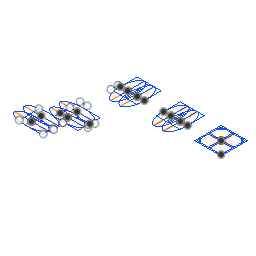
Plano_Apoyos v6 (Autodesk Fusion 360 design; units mm, degrees)
Autodesk Fusion 360 part; units mm, degrees
sketch "V1" plane through (0, 0, 0) normal (0, 1, 0) x (1, 0, 0)
  line L0 (10, -15) -> (10, -28)
  line L1 (10, -28) -> (10, -43)
  line L2 (10, -43) -> (10, -56)
  line L3 (60, -56) -> (60, -43)
  line L4 (60, -43) -> (60, -28)
  line L5 (60, -28) -> (60, -15)
  line L6 (64.9198, -28) -> (64.9198, -34)
  line L7 (64.9198, -34) -> (64.9198, -37)
  line L8 (64.9198, -37) -> (64.9198, -43)
  line L9 (60, -34) -> (35, -34)
  line L10 (35, -34) -> (35, -37)
  line L11 (35, -37) -> (60, -37)
  line L12 (60, -131, 30) -> (60, -118, 30)
  line L13 (60, -118, 30) -> (60, -103, 30)
  line L14 (60, -103, 30) -> (60, -90, 30)
  line L15 (10, -90, 30) -> (10, -103, 30)
  line L16 (10, -103, 30) -> (10, -118, 30)
  line L17 (10, -118, 30) -> (10, -131, 30)
  line L18 (60, -109, 30) -> (35, -109, 30)
  line L19 (35, -112, 30) -> (60, -112, 30)
  line L20 (35, -109, 30) -> (35, -112, 30)
  line L21 (35, -109, 30) -> (10, -109, 30)
  line L22 (35, -112, 30) -> (10, -112, 30)
  line L23 (60, -15) -> (60, -12.5)
  line L24 (60, -12.5) -> (10, -12.5)
  line L25 (10, -12.5) -> (10, -15)
  line L26 (10, -56) -> (10, -58.5)
  line L27 (10, -58.5) -> (60, -58.5)
  line L28 (60, -58.5) -> (60, -56)
  line L29 (60, -25.5) -> (10, -25.5)
  line L30 (60, -45.5) -> (10, -45.5)
  line L31 (10, -4.3386) -> (25, -4.3386)
  ellipse E0 centre (25, -25.5) end of major axis (60, -25.5) minor radius 13
  line L32 (-10, -25.5) -> (60, -25.5)
  line L33 (25, -38.5) -> (25, -12.5)
  ellipse E1 centre (25, -45.5) end of major axis (60, -45.5) minor radius 13
  line L34 (-10, -45.5) -> (60, -45.5)
  line L35 (25, -58.5) -> (25, -32.5)
  line L36 (60, -90, 30) -> (60, -87.5, 30)
  line L37 (60, -87.5, 30) -> (10, -87.5, 30)
  line L38 (10, -87.5, 30) -> (10, -90, 30)
  line L39 (10, -131, 30) -> (10, -133.5, 30)
  line L40 (10, -133.5, 30) -> (60, -133.5, 30)
  line L41 (60, -133.5, 30) -> (60, -131, 30)
  line L42 (60, -109, 30) -> (63, -109, 30)
  line L43 (63, -109, 30) -> (63, -100.5, 30)
  line L44 (63, -100.5, 30) -> (60, -100.5, 30)
  line L45 (60, -112, 30) -> (63, -112, 30)
  line L46 (63, -112, 30) -> (63, -120.5, 30)
  line L47 (63, -120.5, 30) -> (60, -120.5, 30)
  line L48 (60, -100.5, 30) -> (10, -100.5, 30)
  line L49 (60, -120.5, 30) -> (10, -120.5, 30)
  curve E2
  line L50 (-10, -100.5, 30) -> (60, -100.5, 30)
  line L51 (25, -113.5, 30) -> (25, -87.5, 30)
  curve E3
  line L52 (-10, -120.5, 30) -> (60, -120.5, 30)
  line L53 (25, -133.5, 30) -> (25, -107.5, 30)
  point P0 (60, -34)
  point P1 (10, -45.5)
  point P2 (25, -25.5)
  point P3 (25, -45.5)
  point P4 (25, -100.5)
  point P5 (25, -120.5)
  dimension "d4" = 50
  dimension "d9" = 3
  dimension "d25" = 8.5
  dimension "d26" = 8.5
  dimension "d28" = 20
  dimension "d32" = 8.5
  dimension "d33" = 8.5
  dimension "d47" = 13
  constraint coincident L4 P0
  constraint perpendicular L4 L9
  constraint perpendicular L9 L10
  constraint perpendicular L4 L11
  constraint perpendicular L5 L24
  constraint coincident L3 L30.start
  constraint coincident L5 L29.start
  constraint coincident P0 L9.start
  constraint coincident L29.start L32.end
  constraint perpendicular L5 L29
  constraint coincident L30.start L34.end
  constraint coincident L2 P1
  constraint perpendicular L2 L30
  constraint coincident P1 L30.end
  constraint perpendicular L25 L31
  constraint coincident L24 L33.end
  constraint coincident L29 P2
  constraint coincident L30 P3
  constraint coincident L27 L35.start
  constraint coincident P2 E0.centre
  constraint perpendicular L5 L32
  constraint coincident E0 L32.start
  constraint coincident L29.start E0
  constraint coincident E0 L33.start
  constraint coincident L33.end E0
  constraint coincident P3 E1.centre
  constraint perpendicular L3 L34
  constraint coincident E1 L34.start
  constraint coincident L30.start E1
  constraint coincident L35.start E1
  constraint coincident E1 L35.end
  measures "d4" distance of L2.end L3.start
  measures "d9" distance of L6.end L7.end
  measures "d25" distance of L11.end L30.start
  measures "d26" distance of L29.start P0
  measures "d28" distance of L29.end P1
  measures "d47" distance of L23.end L29.start
sketch "V2" plane through (0, 0, 0) normal (0, 1, 0) x (1, 0, 0)
  line L0 (25, 50) -> (40, 50)
  line L1 (40, 50) -> (48.5, 50)
  line L2 (48.5, 50) -> (51.5, 50)
  line L3 (51.5, 50) -> (60, 50)
  line L4 (60, 50) -> (75, 50)
  line L5 (75, 50) -> (75, 100)
  line L6 (75, 100) -> (60, 100)
  line L7 (60, 100) -> (51.5, 100)
  line L8 (51.5, 100) -> (48.5, 100)
  line L9 (48.5, 100) -> (40, 100)
  line L10 (40, 100) -> (25, 100)
  line L11 (25, 100) -> (25, 50)
  line L12 (60, 50) -> (60, 100)
  line L13 (40, 50) -> (40, 100)
  line L14 (48.5, 50) -> (48.5, 75)
  line L15 (48.5, 75) -> (48.5, 100)
  line L16 (51.5, 50) -> (51.5, 75)
  line L17 (51.5, 75) -> (51.5, 100)
  line L18 (20.0289, 50) -> (20.0289, 65)
  ellipse E0 centre (40, 65) end of major axis (40, 100) minor radius 15
  line L19 (40, 30) -> (40, 100)
  line L20 (55, 65) -> (25, 65)
  ellipse E1 centre (60, 65) end of major axis (60, 100) minor radius 15
  line L21 (60, 30) -> (60, 100)
  line L22 (75, 65) -> (45, 65)
  line L23 (51.5, 75) -> (48.5, 75)
  line L24 (138.5, 50) -> (138.5, 75)
  line L25 (141.5, 50) -> (141.5, 75)
  line L26 (150, 30) -> (150, 100) construction
  ellipse E2 centre (150, 65) end of major axis (150, 100) minor radius 15
  line L27 (150, 30) -> (150, 100)
  line L28 (165, 65) -> (135, 65)
  line L29 (138.5, 75) -> (138.5, 100)
  line L30 (130, 50) -> (130, 100)
  line L31 (141.5, 75) -> (141.5, 100)
  line L32 (141.5, 100) -> (138.5, 100)
  line L33 (165, 50) -> (165, 100)
  line L34 (165, 100) -> (150, 100)
  line L35 (165, 65) -> (135, 65) construction
  line L36 (130, 50) -> (138.5, 50)
  line L37 (141.5, 50) -> (150, 50)
  line L38 (150, 50) -> (165, 50)
  line L39 (141.5, 75) -> (138.5, 75)
  line L40 (138.5, 100) -> (130, 100)
  line L41 (115, 50) -> (130, 50)
  line L42 (130, 100) -> (115, 100)
  line L43 (150, 50) -> (150, 100)
  ellipse E3 centre (130, 65) end of major axis (130, 100) minor radius 15
  line L44 (130, 30) -> (130, 100)
  line L45 (145, 65) -> (115, 65)
  line L46 (138.5, 50) -> (141.5, 50)
  line L47 (150, 100) -> (141.5, 100)
  line L48 (115, 100) -> (115, 50)
  line L49 (145, 65) -> (115, 65) construction
  line L50 (130, 30) -> (130, 100) construction
  line L51 (200, 100) -> (255, 100)
  line L52 (255, 100) -> (255, 45)
  line L53 (255, 45) -> (200, 45)
  line L54 (200, 45) -> (200, 100)
  line L55 (252.5, 47.5) -> (202.5, 47.5)
  line L56 (202.5, 47.5) -> (202.5, 97.5)
  line L57 (202.5, 97.5) -> (252.5, 97.5)
  line L58 (252.5, 97.5) -> (252.5, 47.5)
  line L59 (202.5, 74) -> (252.5, 74)
  line L60 (252.5, 74) -> (252.5, 71)
  line L61 (252.5, 71) -> (202.5, 71)
  line L62 (202.5, 71) -> (202.5, 74)
  line L63 (202.5, 74) -> (252.5, 71) construction
  line L64 (252.5, 74) -> (202.5, 71) construction
  line L65 (229, 97.5) -> (226, 97.5)
  line L66 (226, 97.5) -> (226, 47.5)
  line L67 (226, 47.5) -> (229, 47.5)
  line L68 (229, 47.5) -> (229, 97.5)
  line L69 (229, 97.5) -> (226, 47.5) construction
  line L70 (226, 97.5) -> (229, 47.5) construction
  line L71 (202.5, 47.5) -> (202.5, 55.5)
  line L72 (202.5, 47.5) -> (210.5, 47.5)
  line L73 (202.5, 55.5) -> (210.5, 47.5)
  line L74 (202.5, 55.5) -> (200, 55.5)
  line L75 (210.5, 47.5) -> (210.5, 45)
  line L76 (210.5, 45) -> (200, 55.5)
  line L77 (255, 55.5) -> (244.5, 45)
  line L78 (244.5, 47.5) -> (244.5, 45)
  line L79 (244.5, 47.5) -> (252.5, 55.5)
  line L80 (252.5, 55.5) -> (255, 55.5)
  line L81 (244.5, 100) -> (255, 89.5)
  line L82 (252.5, 89.5) -> (255, 89.5)
  line L83 (252.5, 89.5) -> (244.5, 97.5)
  line L84 (244.5, 97.5) -> (244.5, 100)
  line L85 (200, 89.5) -> (210.5, 100)
  line L86 (210.5, 97.5) -> (210.5, 100)
  line L87 (210.5, 97.5) -> (202.5, 89.5)
  line L88 (202.5, 89.5) -> (200, 89.5)
  point P0 (25, 65)
  point P1 (40, 65)
  point P2 (60, 65)
  point P3 (75, 65)
  point P4 (130, 65)
  point P5 (150, 65)
  point P6 (165, 65)
  point P7 (115, 65)
  point P8 (252.5, 47.5)
  point P9 (227.5, 72.5)
  point P10 (227.5, 72.5)
  point P11 (227.5, 72.5)
  dimension "d56" = 50
  dimension "d57" = 15
  dimension "d58" = 8.5
  dimension "d59" = 3
  dimension "d60" = 8.5
  dimension "d61" = 15
  dimension "d64" = 25
  dimension "d65" = 15
  dimension "d66" = 50
  dimension "d67" = 15
  dimension "d68" = 8.5
  dimension "d69" = 3
  dimension "d70" = 8.5
  dimension "d71" = 15
  dimension "d72" = 25
  dimension "d73" = 55
  dimension "d78" = 50
  dimension "d80" = 3
  dimension "d83" = 3
  dimension "d84" = 8
  dimension "d85" = 8
  dimension "d87" = 360
  constraint horizontal L0
  constraint parallel L0 L1
  constraint parallel L0 L2
  constraint parallel L0 L3
  constraint parallel L3 L4
  constraint perpendicular L4 L5
  constraint perpendicular L5 L6
  constraint perpendicular L5 L7
  constraint parallel L7 L8
  constraint parallel L8 L9
  constraint parallel L8 L10
  constraint perpendicular L9 L14
  constraint perpendicular L8 L16
  constraint perpendicular L0 L18
  constraint coincident L11 P0
  constraint coincident L13 P1
  constraint coincident L12 P2
  constraint coincident L5 P3
  constraint coincident P1 E0.centre
  constraint parallel L13 L19
  constraint coincident E0 L19.start
  constraint coincident L9.end E0
  constraint coincident E0 L20.start
  constraint coincident E0 P0
  constraint coincident P2 E1.centre
  constraint parallel L12 L21
  constraint coincident E1 L21.start
  constraint coincident L6.end E1
  constraint coincident E1 P3
  constraint coincident E1 L22.end
  constraint perpendicular L16 L23
  constraint horizontal L41
  constraint parallel L36 L41
  constraint parallel L41 L46
  constraint parallel L37 L41
  constraint parallel L37 L38
  constraint perpendicular L33 L38
  constraint perpendicular L33 L34
  constraint perpendicular L33 L47
  constraint parallel L32 L47
  constraint parallel L32 L40
  constraint parallel L32 L42
  constraint perpendicular L24 L40
  constraint perpendicular L25 L32
  constraint coincident P7 L48
  constraint coincident P4 L30
  constraint coincident P5 L43
  constraint coincident P6 L33
  constraint coincident P4 E3.centre
  constraint parallel L30 L44
  constraint coincident L44.start E3
  constraint coincident L30.end E3
  constraint coincident L45.start E3
  constraint coincident P7 E3
  constraint coincident P5 E2.centre
  constraint parallel L26 L43
  constraint coincident L26.start E2
  constraint coincident L26.end E2
  constraint coincident P6 E2
  constraint coincident L28.end E2
  constraint perpendicular L25 L39
  constraint horizontal L51
  constraint vertical L52
  constraint horizontal L53
  constraint vertical L54
  constraint horizontal L55
  constraint vertical L56
  constraint horizontal L57
  constraint vertical L58
  constraint coincident P8 L55.start
  constraint perpendicular L59 L60
  constraint parallel L59 L61
  constraint parallel L60 L62
  constraint horizontal L59
  constraint coincident L63 P11
  constraint coincident L64 P11
  constraint coincident P11 P10
  constraint perpendicular L65 L66
  constraint parallel L65 L67
  constraint parallel L66 L68
  constraint horizontal L65
  constraint coincident L69 P11
  constraint coincident L70 P11
  constraint perpendicular L55 L71
  constraint perpendicular L56 L72
  constraint coincident L54 L74.end
  constraint perpendicular L54 L74
  constraint coincident L53 L75.end
  constraint perpendicular L53 L75
  constraint parallel L73 L76
  measures "d56" distance of L4.end L5.end
  measures "d57" distance of L3.end L4.end
  measures "d58" distance of L2.end L3.end
  measures "d59" distance of L1.end L2.end
  measures "d60" distance of L0.end L1.end
  measures "d61" distance of L0.start L0.end
  measures "d64" distance of L2.end L16.end
  measures "d65" distance of L18.start L18.end
  measures "d66" distance of L33.start L33.end
  measures "d67" distance of L37.end L33.start
  measures "d68" distance of L37.end L25.start
  measures "d69" distance of L24.start L25.start
  measures "d70" distance of L30.start L24.start
  measures "d71" distance of L30.start L41.start
  measures "d72" distance of L25.end L25.start
  measures "d73" distance of L51.start L51.end
  measures "d78" distance of P8 L57.end
  measures "d80" distance of L59.end L60.end
  measures "d83" distance of L66.end L67.end
  measures "d84" distance of L55.end L71.end
  measures "d85" distance of L55.end L72.end
extrude "Extrude5" add sketch "V2" along normal blind 3 contours L0 L11 E0 | L0 L13 E0 L19 L20 | L13 E0 L19 L20 | L1 L13 L19 L20 E1 | L13 L15 E0 L19 L20 E1 | L9 L15 E0 | L1 L14 L20 E1 L22 | L8 L15 L17 E0 E1 | L15 E0 E1 | L14 L15 L20 E1 L22 | L3 L12 E0 L21 L22 | L3 L16 E0 L20 L22 | L7 L17 E1 | L15 L17 E0 E1 L23 | L17 E0 E1 | L4 L12 E1 L21 L22 | L16 L17 E0 L20 L22 | L12 L17 E0 E1 L21 L22 | L4 L5 E1 | L12 E1 L21 L22 makes body 1
extrude "Extrude6" add sketch "V2" along normal blind 3 separate body contours L24 E2 L28 L36 L45 | L24 L25 L28 L45 L46 | L24 E2 L28 L29 L45 | L24 L25 L28 L39 L45 | E2 L30 L36 L44 L45 | L25 L28 L37 E3 L45 | L25 L28 L31 E3 L45 | E2 L29 L30 E3 L44 L45 | L30 L41 E3 L44 L45 | L27 L28 L37 L43 E3 | E2 L27 L28 L31 L43 E3 | L30 E3 L44 L45 | L41 E3 L48 | E2 L27 L28 L38 L43 | L29 L40 E3 | E2 L27 L28 L43 | E2 L33 L38 | E2 L31 L47 makes body 2
extrude "Extrude7" add sketch "V2" along normal blind 3 separate body contours L57 L85 L86 | L51 L57 L65 L84 L86 | L54 L56 L62 L74 L88 | L56 L85 L88 | L57 L81 L84 | L56 L57 L85 L87 | L56 L57 L59 L66 L87 | L56 L71 L74 L76 | L57 L58 L81 L83 | L57 L58 L59 L68 L83 | L55 L56 L71 L72 L73 L76 | L55 L56 L61 L66 L73 | L58 L81 L82 | L52 L58 L60 L80 L82 | L53 L55 L67 L75 L78 | L55 L72 L75 L76 | L58 L77 L80 | L55 L77 L78 | L55 L58 L77 L79 | L55 L58 L61 L68 L79 makes body 3
copy_body "Body->Comp5" bodies 1 removing the originals makes body 4 in component "Apoyo_A"
copy_body "Body->Comp6" bodies 2 removing the originals makes body 5 in component "Apoyo_B"
copy_body "Body->Comp7" bodies 3 removing the originals makes body 6 in component "Base_Apoyo "
extrude "Extrude3" [suppressed]
extrude "Extrude4" [suppressed]
copy_body "Body->Comp3" [suppressed] in component "Apoyo1"
copy_body "Body->Comp4" [suppressed] in component "Apoyo2"
component "Apoyo_A" placed x (1, 0, 0) y (0, 1, 0) z (0, 0, 1) at (0, 0, 0)
component "Apoyo_B" placed x (1, 0, 0) y (0, 1, 0) z (0, 0, 1) at (0, 0, 0)
component "Base_Apoyo " placed x (1, 0, 0) y (0, 1, 0) z (0, 0, 1) at (0, 0, 0)
equation "d25 = ( 17 / 2 ) * 1 mm"
equation "d26 = ( 17 / 2 ) * 1 mm"
equation "d32 = ( 17 / 2 ) * 1 mm"
named bodies: "Apoyo_A", "Apoyo_B", "Base_Apoyo"
